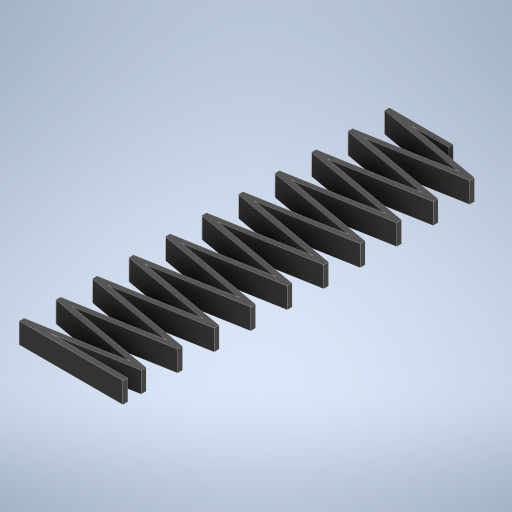
# Autodesk Inventor part: spring
Saved by Autodesk Inventor 2024.1 (Build 281209000, 209)
## iProperties
Created: 2024-11-06
Part Number: spring
Material: 鉛
Document SubType Name: Modeling
Designer: hibik
Density: 11.34 g/cm^3
Appearance: 鉛
Author: hibik
Autodesk Inventor part; units mm, degrees
ref_plane "YZ Plane" through (0, 0, 0) normal (1, 0, 0) x (0, 1, 0)
ref_plane "XZ Plane" through (0, 0, 0) normal (0, 1, 0) x (-1, 0, 0)
ref_plane "XY Plane" through (0, 0, 0) normal (0, 0, 1) x (1, 0, 0)
sketch "スケッチ2" plane through (0, 0, 0) normal (0, 1, 0) x (-1, 0, 0)
  line L0 (32.5, 0) -> (-32.5, 0)
  line L1 (-32.5, 0) -> (-32.5, -3)
  line L2 (-32.5, -3) -> (32.5, -3)
  line L3 (32.5, -3) -> (32.5, 0)
  point P0 (0, 0)
  point P1 (0, 0)
  dimension "d8" = 65
  dimension "d9" = 3
  constraints: 8 end point, 2 parallel, 1 coincident, 1 horizontal, 1 midpoint, 1 perpendicular
  measures "d8" distance of L2.end L1.end
  measures "d9" distance of L0.end L1.end
extrude "押し出し2" add sketch "スケッチ2" along normal blind 13
sketch "スケッチ3" plane through (0, 0, 0) normal (0, -1, 0) x (1, 0, 0)
  line L0 (-32.2395, -0.0228) -> (-32.7605, -2.9772) construction
  line L1 (-32.7605, -2.9772) -> (32.2395, -14.4385)
  line L2 (32.2395, -14.4385) -> (32.7605, -11.484) construction
  line L3 (32.7605, -11.484) -> (-32.2395, -0.0228)
  line L4 (32.2395, -11.484) -> (32.7605, -14.4385) construction
  line L5 (32.7605, -14.4385) -> (-32.2395, -25.8997)
  line L6 (-32.2395, -25.8997) -> (-32.7605, -22.9453) construction
  line L7 (-32.7605, -22.9453) -> (32.2395, -11.484)
  line L8 (-32.5, -3) -> (-32.5, 0) projected
  line L9 (32.5, -3) -> (-32.5, -3) projected
  line L10 (32.5, 0) -> (32.5, -3) projected
  line L11 (-32.5, 0) -> (-32.5, -3.0231)
  line L12 (-32.2395, -25.8997) -> (-32.2395, -22.8534)
  line L13 (32.5, -11.4381) -> (32.5, -14.4844)
  line L14 (-32.5, -3) -> (-32.5, 0) projected
  line L15 (-32.2395, -0.0228) -> (-32.5, 0)
  point P0 (32.5, -12.9613)
  point P1 (-32.5, -1.5)
  point P2 (-32.5, -1.5)
  point P3 (-32.5, -24.4225)
  point P4 (32.5, -1.5)
  point P5 (-15.3549, -3)
  point P6 (23.8618, -12.9613)
  point P7 (-32.2395, -24.3766)
  point P8 (-32.5, -1.5)
  dimension "d13" = 10
  dimension "d14" = 20
  dimension "d17" = 22.8766
  constraints: 24 end point, 10 midpoint, 5 point on line, 4 parallel, 2 equal length, 2 perpendicular, 2 vertical, 2 vertical alignment
  measures "d13" angle of L9 L3
  measures "d14" angle of L7 L1
  measures "d17" vertical distance of point (-32.24, -24.377) point (-32.5, -1.5)
extrude "押し出し3" add sketch "スケッチ3" against normal up to surface (13 mm away)
pattern_linear "矩形状パターン1" count 10 spacing 22.877 along (0, 0, -1) of "押し出し3"
sketch "スケッチ4" plane through (0, 0, 0) normal (0, -1, 0) x (1, 0, 0)
  line L0 (32.7605, -228.7696) -> (-32.2395, -228.7696)
  line L1 (-32.2395, -228.7696) -> (-32.2395, -231.7696)
  line L2 (-32.2395, -231.7696) -> (32.7605, -231.7696)
  line L3 (32.7605, -231.7696) -> (32.7605, -228.7696)
  line L4 (-32.5, 0) -> (32.5, 0) projected
  line L5 (-32.2395, -228.7464) -> (-32.2395, -231.7927) projected
  line L6 (32.5, -3) -> (-15.3549, -3) projected
  point P0 (0, 0)
  point P1 (-32.2395, -230.2696)
  dimension "d21" = 3
  dimension "d24" = 3
  constraints: 8 end point, 3 parallel, 2 midpoint, 1 horizontal, 1 perpendicular
  measures "d21" distance of L1.end L0.end
  measures "d24" distance between parallel lines of L6 L4
extrude "押し出し4" add sketch "スケッチ4" against normal up to surface (13 mm away)
sketch "スケッチ5" plane through (0, 13, 0) normal (0, 1, 0) x (1, 0, 0)
  line L0 (32.7605, 228.7696) -> (7.7605, 228.7696)
  line L1 (7.7605, 228.7696) -> (7.7605, 231.7696)
  line L2 (7.7605, 231.7696) -> (32.7605, 231.7696)
  line L3 (32.7605, 231.7696) -> (32.7605, 228.7696)
  line L4 (32.7605, 231.7696) -> (32.7605, 228.7696) projected
  line L5 (32.7605, 228.7696) -> (-15.0944, 228.7696) projected
  line L6 (-32.1083, 231.7696) -> (32.7605, 231.7696) projected
  point P0 (0, 0)
  dimension "d25" = 25
  constraints: 8 end point, 3 collinear, 2 parallel, 1 horizontal, 1 perpendicular
  measures "d25" distance between parallel lines of L4 L1
extrude "押し出し5" cut sketch "スケッチ5" against normal through all
equation "\"d13\" = 0.5 * d14"
equation "\"d21\" = d24"
